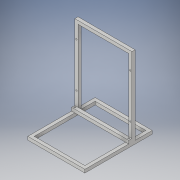
# Autodesk Inventor part: Test stand v1.2
Saved by Autodesk Inventor 2019 (Build 230136000, 136)
## iProperties
Created: 2021-03-22
Part Number: Test stand v1.2
Material: Generic
Document SubType Name: Modeling
Designer: User
Density: 1 g/cm^3
Appearance: Default
Author: User
Autodesk Inventor part; units mm, degrees
ref_plane "YZ Plane" through (0, 0, 0) normal (1, 0, 0) x (0, 1, 0)
ref_plane "XZ Plane" through (0, 0, 0) normal (0, 1, 0) x (-1, 0, 0)
ref_plane "XY Plane" through (0, 0, 0) normal (0, 0, 1) x (1, 0, 0)
sketch "Sketch1" plane through (0, 0, 0) normal (0, 1, 0) x (-1, 0, 0)
  line L0 (0, 0) -> (297, 0)
  line L1 (297, 0) -> (297, -357)
  line L2 (297, -357) -> (0, -357)
  line L3 (0, -357) -> (0, 0)
  line L4 (-19, 19) -> (316, 19)
  line L5 (316, 19) -> (316, -376)
  line L6 (316, -376) -> (-19, -376)
  line L7 (-19, -376) -> (-19, 19)
  dimension "d2" = 19
  dimension "d3" = 19
  dimension "d4" = 19
  dimension "d5" = 19
  dimension "d6" = 395
  dimension "d7" = 335
  constraints: 16 end point, 4 parallel, 2 horizontal, 2 perpendicular
  measures "d2" distance between parallel lines of L5 L1
  measures "d3" distance between parallel lines of L2 L6
  measures "d4" distance between parallel lines of L3 L7
  measures "d5" distance between parallel lines of L0 L4
  measures "d6" distance between parallel lines of L6 L4
  measures "d7" distance between parallel lines of L7 L5
extrude "Extrusion1" add sketch "Sketch1" along normal mid plane 19
sketch "Sketch3" plane through (0, 9.5, 0) normal (0, 1, 0) x (1, 0, 0)
  line L0 (-316, 376) -> (-316, -19) projected
  line L1 (-316, 276) -> (-297, 276)
  line L2 (-297, 276) -> (-297, 257)
  line L3 (-297, 257) -> (-316, 257)
  line L4 (-316, 257) -> (-316, 276)
  line L5 (0, 357) -> (0, 0) projected
  line L6 (19, 376) -> (19, -19) projected
  line L7 (0, 276) -> (19, 276)
  line L8 (19, 276) -> (19, 257)
  line L9 (19, 257) -> (0, 257)
  line L10 (0, 257) -> (0, 276)
  line L11 (19, 376) -> (-316, 376) projected
  dimension "d26" = 19
  dimension "d27" = 19
  dimension "d28" = 100
  constraints: 16 end point, 5 point on line, 4 parallel, 2 horizontal, 2 perpendicular
  measures "d26" distance between parallel lines of L0 L2
  measures "d27" distance between parallel lines of L9 L7
  measures "d28" distance between parallel lines of L1 L11
extrude "Extrusion2" add sketch "Sketch3" along normal blind 460
sketch "Sketch4" plane through (-297, -9.5, 0) normal (1, 0, 0) x (0, 0, -1)
  line L0 (257, 19) -> (257, 479) projected
  line L1 (276, 19) -> (276, 479) projected
  line L2 (257, 479) -> (276, 479)
  line L3 (276, 479) -> (276, 460)
  line L4 (276, 460) -> (257, 460)
  line L5 (257, 460) -> (257, 479)
  point P0 (0, 9.5)
  dimension "d31" = 19
  constraints: 8 end point, 2 parallel, 1 horizontal, 1 perpendicular, 1 point on line
  measures "d31" distance between parallel lines of L4 L2
extrude "Extrusion3" add sketch "Sketch4" along normal blind 316
sketch "Sketch5" plane through (19, 469.5, -276) normal (0, 0, -1) x (-1, 0, 0)
  circle A0 centre (9.5, -100) radius 4
  circle A1 centre (325.5, -100) radius 4
  circle A2 centre (9.5, -360) radius 4
  circle A3 centre (325.5, -360) radius 4
  line L0 (335, -460) -> (335, 0) projected
  line L1 (0, 0) -> (335, 0) projected
  line L2 (19, -460) -> (19, -19) projected
  line L3 (0, -460) -> (335, -460) projected
  line L4 (0, -460) -> (0, 0) projected
  point P0 (19, -469.5)
  dimension "d34" = 8
  dimension "d35" = 8
  dimension "d36" = 8
  dimension "d37" = 8
  dimension "d38" = 9.5
  dimension "d39" = 100
  dimension "d40" = 100
  dimension "d41" = 9.5
  dimension "d42" = 9.5
  dimension "d43" = 100
  dimension "d44" = 100
  dimension "d45" = 9.5
  constraints: 4 centre point
  measures "d34" diameter of A0
  measures "d35" diameter of A1
  measures "d36" diameter of A2
  measures "d37" diameter of A3
  measures "d38" distance from line of L0 A1.centre
  measures "d39" distance from line of A0.centre L1
  measures "d40" distance from line of L1 A1.centre
  measures "d41" distance from line of L2 A2.centre
  measures "d42" distance from line of L0 A3.centre
  measures "d43" distance from line of L3 A2.centre
  measures "d44" distance from line of L3 A3.centre
  measures "d45" distance from line of L4 A0.centre
extrude "Extrusion4" cut sketch "Sketch5" against normal blind 19 contours A0 | A1 | A2 | A3
sketch "Sketch6" plane through (0, 9.5, 0) normal (0, 1, 0) x (1, 0, 0)
  line L0 (19, 376) -> (19, -19) projected
  line L1 (-316, 257) -> (19, 257)
  line L2 (19, 257) -> (19, 238)
  line L3 (19, 238) -> (-316, 238)
  line L4 (-316, 238) -> (-316, 257)
  line L5 (19, 376) -> (-316, 376) projected
  point P0 (0, 0)
  dimension "d48" = 19
  dimension "d49" = 335
  dimension "d51" = 119
  constraints: 8 end point, 2 parallel, 1 horizontal, 1 perpendicular, 1 point on line
  measures "d48" distance between parallel lines of L1 L3
  measures "d49" distance between parallel lines of L4 L0
  measures "d51" distance between parallel lines of L5 L1
extrude "Extrusion5" add sketch "Sketch6" along normal blind 19
sketch "Sketch7" plane through (0, 28.5, 0) normal (0, 1, 0) x (1, 0, 0)
  circle A0 centre (-306.5, 247.5) radius 4
  circle A1 centre (9.5, 247.5) radius 4
  line L0 (19, 238) -> (19, 257) projected
  line L1 (-316, 238) -> (19, 238) projected
  line L2 (-316, 257) -> (-316, 238) projected
  point P0 (0, 0)
  dimension "d54" = 8
  dimension "d55" = 8
  dimension "d56" = 9.5
  dimension "d57" = 9.5
  dimension "d58" = 9.5
  dimension "d59" = 9.5
  constraints: 2 centre point
  measures "d54" diameter of A0
  measures "d55" diameter of A1
  measures "d56" distance from line of L0 A1.centre
  measures "d57" distance from line of A1.centre L1
  measures "d58" distance from line of L2 A0.centre
  measures "d59" distance from line of L1 A0.centre
extrude "Extrusion6" cut sketch "Sketch7" against normal blind 39
body "Solid1"
